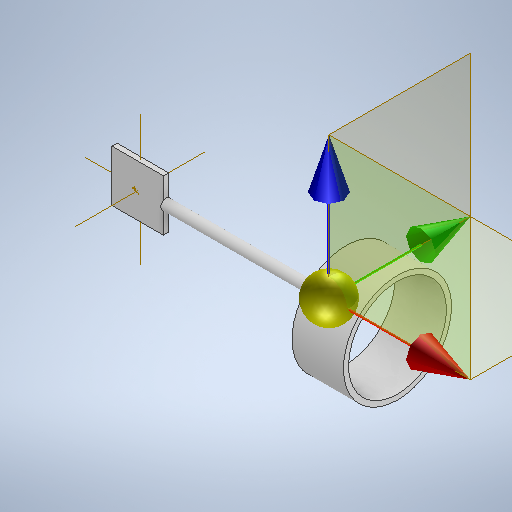
# Autodesk Inventor part: EAO Test Ref
Saved by Autodesk Inventor 2025 (Build 290162010, 162A)
## iProperties
Created: 2025-01-30
Part Number: EAO Test Ref
Material: Generic
Document SubType Name: Modeling
Designer: paulj
Mass: 838274 g
Surface Area: 184467 cm^2
Volume: 838274 cm^3
Density: 1 g/cm^3
Appearance: Default
Author: paulj
Autodesk Inventor part; units mm, degrees
ref_plane "YZ Plane" through (0, 0, 0) normal (1, 0, 0) x (0, 1, 0)
ref_plane "XZ Plane" through (0, 0, 0) normal (0, 1, 0) x (-1, 0, 0)
ref_plane "XY Plane" through (0, 0, 0) normal (0, 0, 1) x (1, 0, 0)
sketch "Sketch3" plane through (0, 0, 0) normal (0, 1, 0) x (-1, 0, 0)
  line L0 (-500, -500) -> (500, -500)
  line L1 (500, -500) -> (500, 500)
  line L2 (500, 500) -> (-500, 500)
  line L3 (-500, 500) -> (-500, -500)
  line L4 (-500, -500) -> (500, 500) construction
  line L5 (500, -500) -> (-500, 500) construction
  point P0 (0, 0)
  dimension "d8" = 1000
  dimension "d9" = 1000
  constraints: 12 end point, 2 midpoint, 2 parallel, 1 horizontal, 1 perpendicular
  measures "d8" distance of L2.end L1.end
  measures "d9" distance of L1.end L0.end
extrude "Extrusion3" add sketch "Sketch3" along normal mid plane 100
sketch "Sketch4" plane through (500, -50, -500) normal (1, 0, 0) x (0, 0, -1)
  circle A0 centre (-500, 50) radius 100
  dimension "d12" = 100
  constraints: 1 centre point, 1 coincident
  measures "d12" radius of A0
extrude "Extrusion4" add sketch "Sketch4" along normal blind 3500
sketch "Sketch6" plane through (4000, 0, 0) normal (1, 0, 0) x (0, 0, -1)
  circle A0 centre (0, 0) radius 1000 construction
  circle A1 centre (0, 0) radius 1050
  circle A2 centre (0, 0) radius 950
  dimension "d18" = 1000
  dimension "d21" = 50
  dimension "d22" = 50
  constraints: 3 centre point, 3 coincident
  measures "d18" radius of A0
  measures "d21" radial gap between concentric circles of A0 A2
  measures "d22" radial gap between concentric circles of A1 A0
extrude "Extrusion6" add sketch "Sketch6" along normal blind 1000
body "Solid1"
body "Solid2"
